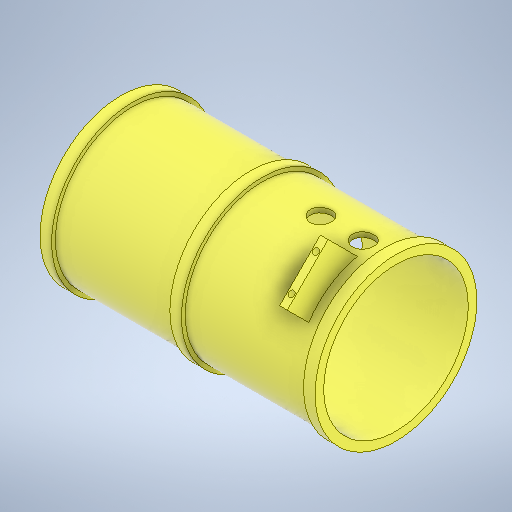
# Autodesk Inventor part: 1 part 28
Saved by Autodesk Inventor 2025.1 (Build 291241000, 241)
## iProperties
Created: 2024-08-01
Part Number: 1 part 28
Material: Steel, Alloy
Document SubType Name: Modeling
Designer: ffogue
Density: 7.73 g/cm^3
Appearance: Smooth - Yellow
Author: ffogue
Autodesk Inventor part; units mm, degrees
sketch "Sketch2" plane through (0, 0, 0) normal (0, 0, 1) x (1, 0, 0)
  line L0 (0, 0) -> (0, 42)
  line L1 (0, 42) -> (6, 42)
  line L2 (6, 42) -> (6, 40)
  line L3 (6, 40) -> (67.5, 40)
  line L4 (67.5, 40) -> (67.5, 42)
  line L5 (67.5, 42) -> (73.5, 42)
  line L6 (73.5, 42) -> (73.5, 40)
  line L7 (73.5, 40) -> (137, 40)
  line L8 (137, 40) -> (137, 42)
  line L9 (137, 42) -> (143, 42)
  line L10 (143, 42) -> (143, 0)
  line L11 (143, 0) -> (0, 0)
  dimension "d4" = 84
  dimension "d6" = 80
  dimension "d7" = 6
  dimension "d8" = 6
  dimension "d9" = 6
  dimension "d10" = 61.5
  dimension "d11" = 63.5
  constraints: 24 end point, 8 perpendicular, 6 point on line, 1 horizontal alignment, 1 vertical
  measures "d4" diameter of L1 L11
  measures "d6" diameter of L3 L11
  measures "d7" distance of L0.end L1.end
  measures "d8" distance of L4.end L5.end
  measures "d9" distance of L8.end L9.end
  measures "d10" distance between parallel lines of L2 L4
  measures "d11" distance between parallel lines of L8 L6
revolve "Revolution1" add sketch "Sketch2" angle 360 about axis through (143, 0, 0) along (-1, 0, 0)
sketch "Sketch3" plane through (143, 0, 0) normal (1, 0, 0) x (0, 0, -1)
  circle A0 centre (0, 0) radius 42 projected
  constraints: 1 coincident
hole "Hole1" at (143, 0, 0) direction (-1, 0, 0) diameter 75 depth 143
ref_plane "Work Plane2" through (0, 40, 0) normal (0, 1, 0) x (-1, 0, 0)
sketch "Sketch5" plane through (0, 40, 0) normal (0, 1, 0) x (-1, 0, 0)
  line L0 (-143, -42) -> (-143, 42) projected
  point P0 (0, 0)
  point P1 (-36, 0)
  point P2 (-81, 0)
  dimension "d31" = 45
  dimension "d32" = 62
  constraints: 2 horizontal alignment
  measures "d31" distance of point (-36, 0) point (-81, 0)
  measures "d32" distance from line of L0 point (-81, 0)
hole "Hole3" at (36, 40, 0) at (81, 40, 0) direction (0, -1, 0) diameter 14 depth 4
ref_plane "Work Plane1" through (0, 0, 40) normal (0, 0, 1) x (1, 0, 0)
sketch "Sketch4" plane through (0, 0, 40) normal (0, 0, 1) x (1, 0, 0)
  line L0 (143, 42) -> (143, -42) projected
  point P0 (0, 0)
  point P1 (126, 0)
  point P2 (104, 0)
  dimension "d21" = 22
  dimension "d22" = 17
  constraints: 2 horizontal alignment
  measures "d21" distance of point (126, 0) point (104, 0)
  measures "d22" distance from line of L0 point (126, 0)
hole "Hole2" at (126, 0, 40) at (104, 0, 40) direction (0, 0, -1) diameter 11 depth 3.5
ref_plane "Work Plane4" through (0, 0, 55) normal (0, 0, 1) x (1, 0, 0)
ref_plane "Work Plane5" through (131.031, 0, 0) normal (-1, 0, 0) x (0, 0, 1)
sketch "Sketch7" plane through (131.031, 0, 0) normal (-1, 0, 0) x (0, 0, 1)
  line L0 (38.8909, -38.8909) -> (-38.8909, 38.8909) construction
  line L1 (0, 0) -> (-55.7325, 0) construction
  dimension "d48" = 45
  dimension "d54" = 110
  constraints: 4 end point, 2 coincident, 2 midpoint, 1 horizontal
  measures "d48" angle of L1 L0
  measures "d54" distance of L0.start L0.end
ref_plane "Work Plane7" through (101.031, 0, 0) normal (-1, 0, 0) x (0, 0, 1)
sketch "Sketch8" plane through (101.031, 0, 0) normal (-1, 0, 0) x (0, 0, 1)
  line L0 (38.8909, -38.8909) -> (-38.8909, 38.8909) construction
  line L1 (0, 0) -> (-62.9991, 0) construction
  dimension "d50" = 45
  dimension "d53" = 110
  constraints: 4 end point, 2 midpoint, 1 coincident, 1 horizontal
  measures "d50" angle of L1 L0
  measures "d53" distance of L0.start L0.end
ref_plane "Work Plane12" through (131.031, -38.8909, 38.8909) normal (0, 0.7071068, -0.7071068) x (-1, 0, 0)
sketch "Sketch10" plane through (131.031, -38.8909, 38.8909) normal (0, 0.7071068, -0.7071068) x (-1, 0, 0)
  line L0 (0, 22) -> (4, 22)
  line L1 (4, 22) -> (4, -8)
  line L2 (4, -8) -> (0, -8)
  line L3 (0, -8) -> (0, 22)
  line L4 (-5.969, -40) -> (57.531, -40) projected
  point P0 (131.031, 0)
  dimension "d55" = 4
  dimension "d56" = 30
  dimension "d59" = 32
  constraints: 8 end point, 2 parallel, 1 horizontal, 1 perpendicular
  measures "d55" distance of L0.start L0.end
  measures "d56" distance of L0.end L1.end
  measures "d59" distance between parallel lines of L4 L2
extrude "Extrusion3" add sketch "Sketch10" along normal up to surface round surface about axis through (105.25, 0, 0) along (-1, 0, 0) radius 40 far side no
sketch "Sketch11" plane through (131.031, -38.8909, 38.8909) normal (0, -0.7071068, 0.7071068) x (1, 0, 0)
  circle A0 centre (-2, 16) radius 1.5
  circle A1 centre (-2, -2) radius 1.5
  line L0 (-4, 22) -> (0, 22) projected
  line L1 (-4, -8) -> (-4, 22) projected
  point P0 (-131.031, 0)
  point P1 (-2, 22)
  point P2 (-4, 7)
  dimension "d60" = 18
  dimension "d61" = 9
  dimension "d62" = 3
  dimension "d63" = 3
  constraints: 2 centre point, 2 midpoint, 2 vertical alignment
  measures "d60" distance of A1.centre A0.centre
  measures "d61" vertical distance of point (-4, 7) A0.centre
  measures "d62" diameter of A0
  measures "d63" diameter of A1
extrude "Extrusion4" cut sketch "Sketch11" against normal up to surface round surface about axis through (105.25, 0, 0) along (-1, 0, 0) radius 40 far side no
equation "\"d8\" = d7"
equation "\"d9\" = d7"
body "Solid2"
